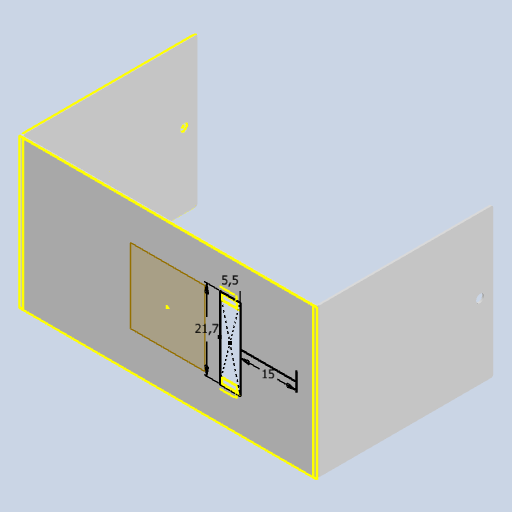
# Autodesk Inventor part: metal_cap
Saved by Autodesk Inventor 2022 (Build 260153000, 153)
## iProperties
Created: 2024-07-26
Part Number: metal_cap
Material: Типовые
Document SubType Name: Sheet Metal
Designer: Капустяник Андрей
Density: 1 g/cm^3
Sheet Metal Rule: По умолчанию
Appearance: По умолчанию
Author: Капустяник Андрей
Autodesk Inventor part; units mm, degrees
ref_plane "YZ Plane" through (0, 0, 0) normal (1, 0, 0) x (0, 1, 0)
ref_plane "XZ Plane" through (0, 0, 0) normal (0, 1, 0) x (-1, 0, 0)
ref_plane "РабПлоскость1" through (0, 0, 24) normal (0, 0, 1) x (1, 0, 0)
sketch "Эскиз1" plane through (0, 0, 24) normal (0, 0, 1) x (1, 0, 0)
  line L0 (-40, 20) -> (40, 20)
  line L1 (40, 20) -> (40, -20)
  line L2 (40, -20) -> (-40, -20)
  line L3 (-40, -20) -> (-40, 20)
  line L4 (-40, 20) -> (40, -20) construction
  line L5 (40, 20) -> (-40, -20) construction
  point P0 (0, 0)
  dimension "d1" = 80
  dimension "d2" = 40
  measures "d1" distance of L1.end L2.end
  measures "d2" distance between parallel lines of L2 L0
extrude "Пластина1" add sketch "Эскиз1" against normal blind 0.5
sketch "Эскиз2" plane through (-39.5, 20, 24) normal (-1, 0, 0) x (0, -1, 0)
  line L0 (40, 0) -> (0, 0)
  line L1 (0, 0) -> (0, -47.5)
  line L2 (0, -47.5) -> (40, -47.5)
  line L3 (40, -47.5) -> (40, 0)
  constraints: 6 end point, 1 horizontal, 1 perpendicular, 1 vertical
edge flange "Фланец1" height 47.5 angle 90 thickness 0.5 bend radius 0.5 thickness toward (-1, 0, 0) relief tear relief width 0.5 relief depth 0.25 corner gap 0.5 corner form 0 edges at (-40, 0, 23.5) (40, 0, 23.5) wall of the first edge with corners at (-39.5, -20, 24) (-39.5, 20, 24) (-39.5, 20, -23.5) (-39.5, -20, -23.5)
bend "Сгиб1"
corner "УглСтык1"
sketch "Эскиз3" plane through (0, 0, 24) normal (0, 0, 1) x (1, 0, 0)
  line L0 (19.5, -10.85) -> (14, -10.85)
  line L1 (14, -10.85) -> (14, 10.85)
  line L2 (14, 10.85) -> (19.5, 10.85)
  line L3 (19.5, 10.85) -> (19.5, -10.85)
  line L4 (19.5, -10.85) -> (14, 10.85) construction
  line L5 (14, -10.85) -> (19.5, 10.85) construction
  line L6 (14.5, -10.5) -> (18.5, -10.5) projected
  line L7 (14.5, -10.5) -> (14.5, -9) projected
  line L8 (18.5, -10.5) -> (18.5, -9) projected
  line L9 (18.5, -9) -> (14.5, -9) projected
  line L10 (14.5, 9) -> (18.5, 9) projected
  line L11 (14.5, 9) -> (14.5, 10.5) projected
  line L12 (14.5, 10.5) -> (18.5, 10.5) projected
  line L13 (18.5, 9) -> (18.5, 10.5) projected
  line L14 (13.98, 11.925) -> (17.88, 11.925) projected
  line L15 (18.38, 10.5) -> (18.38, 11.925) projected
  line L16 (17.88, -11.925) -> (13.98, -11.925) projected
  line L17 (18.38, -11.925) -> (18.38, -10.5) projected
  line L18 (19.5, 9) -> (19.5, -9) projected
  line L19 (19.5, -10.5) -> (19.5, -9) projected
  line L20 (19.5, -10.5) -> (18.5, -10.5) projected
  line L21 (19.5, 9) -> (18.5, 9) projected
  line L22 (34.5, -2.5) -> (34.5, 2.5)
  line L23 (34.5, 0) -> (19.5, 0)
  point P0 (0, 0)
  point P1 (16.75, 0)
  point P2 (14, 0)
  dimension "d14" = 5.5
  dimension "d15" = 21.7
  dimension "d19" = 15
  constraints: 16 end point, 5 midpoint, 2 horizontal, 2 parallel, 1 perpendicular, 1 vertical, 2 other
  measures "d14" distance of L1.end L2.end
  measures "d15" distance of L0.end L1.end
  measures "d19" distance of L23.end L23.start
fillet "УглСкругление1" radius 0.5 4 edges at (-39.75, 20, -23.5) (-39.75, -20, -23.5) (39.75, 20, -23.5) (39.75, -20, -23.5)
extrude "Вырез1" cut sketch "Эскиз3" against normal blind 0.5
sketch "Эскиз4" plane through (-40, -20, 23) normal (-1, 0, 0) x (0, 0, 1)
  circle A0 centre (-43, 20) radius 1.5 projected
  circle A1 centre (-43, 20) radius 1.1
  point P0 (-23, 20)
  dimension "d20" = 2.2
  constraints: 1 centre point, 1 coincident
  measures "d20" diameter of A1
extrude "Вырез2" cut sketch "Эскиз4" against normal blind 80 contours A1
sketch "Эскиз5" plane through (0, 0, 24) normal (0, 0, 1) x (1, 0, 0)
  line L0 (19.5, 10.85) -> (19.5, -10.85) projected
  line L1 (19.5, -10.85) -> (14, -10.85) projected
  line L2 (14, -10.85) -> (14, 10.85) projected
  line L3 (14, 10.85) -> (19.5, 10.85) projected
  line L4 (39, -20) -> (39, 20) projected
  line L5 (-39, 20) -> (39, 20) projected
  line L6 (-39, 20) -> (-39, -20) projected
  line L7 (39, -20) -> (-39, -20) projected
  line L8 (-40, -20) -> (-40, 20) projected
  line L9 (-40, -20) -> (-39, -20) projected
  line L10 (-39, 20) -> (-40, 20) projected
  line L11 (39, -20) -> (40, -20) projected
  line L12 (40, 20) -> (40, -20) projected
  line L13 (40, 20) -> (39, 20) projected
  point P0 (0, 0)
sketch "Эскиз6" plane through (-40, -20, 23) normal (-1, 0, 0) x (0, 0, 1)
  circle A0 centre (-43, 20) radius 1.1 projected
  arc A1 (-46, 40) -> (-46.5, 39.5) centre (-46, 39.5) ccw projected
  line L0 (-46.5, 0.5) -> (-46.5, 39.5) projected
  arc A2 (-46.5, 0.5) -> (-46, 0) centre (-46, 0.5) ccw projected
  line L1 (0, 0) -> (-46, 0) projected
  line L2 (0, 0) -> (0, 40) projected
  line L3 (-46, 40) -> (0, 40) projected
  point P0 (-23, 20)
equation "\"d17\" = Толщина"
equation "\"d3\" = Толщина"
equation "\"d4\" = Ширина_просечки"
equation "\"d5\" = Глубина_просечки"
equation "\"d6\" = Мин_остаток"
equation "\"d7\" = Радиус_перехода"
equation "\"d10\" = Радиус_гибки"
equation "\"d11\" = Размер_просечки"
equation "\"d12\" = Размер_зазора"
equation "\"d13\" = Радиус_Якоби"
equation "\"Радиус_гибки\" = Толщина"
equation "\"Ширина_просечки\" = Толщина"
equation "\"Глубина_просечки\" = 0.5 * Толщина"
equation "\"Размер_просечки\" = 4 * Толщина"
equation "\"Мин_остаток\" = 2 * Толщина"
equation "\"Радиус_перехода\" = Радиус_гибки"
equation "\"Радиус_Якоби\" = Радиус_гибки"
equation "\"Размер_зазора\" = Толщина"
equation "\"Толщина\" = 0.5"
